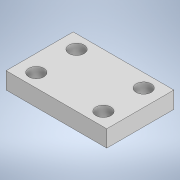
# Autodesk Inventor part: beltpress
Saved by Autodesk Inventor 2020.2 (Build 242310000, 310)
## iProperties
Created: 2020-08-07
Part Number: beltpress
Material: Generic
Document SubType Name: Modeling
Designer: JK
Density: 1 g/cm^3
Appearance: Default
Author: JK
Autodesk Inventor part; units mm, degrees
ref_plane "YZ Plane" through (0, 0, 0) normal (1, 0, 0) x (0, 1, 0)
ref_plane "XZ Plane" through (0, 0, 0) normal (0, 1, 0) x (-1, 0, 0)
ref_plane "XY Plane" through (0, 0, 0) normal (0, 0, 1) x (1, 0, 0)
sketch "Sketch1" plane through (0, 0, 0) normal (0, 1, 0) x (-1, 0, 0)
  line L0 (445.6248, 255.5836) -> (415.6248, 255.5836)
  line L1 (415.6248, 255.5836) -> (415.6248, 235.5836)
  line L2 (415.6248, 235.5836) -> (445.6248, 235.5836)
  line L3 (445.6248, 235.5836) -> (445.6248, 255.5836)
  circle A0 centre (440.6248, 251.5836) radius 2.25
  circle A1 centre (440.6248, 239.5836) radius 2.25
  circle A2 centre (420.6248, 251.5836) radius 2.25
  circle A3 centre (420.6248, 239.5836) radius 2.25
  dimension "d8" = 4.5
  dimension "d9" = 20
  dimension "d10" = 30
  dimension "d11" = 20
  dimension "d12" = 12
  dimension "d13" = 4
  dimension "d14" = 5
  constraints: 8 end point, 4 centre point, 3 equal radius, 2 horizontal alignment, 2 parallel, 2 vertical alignment, 1 horizontal, 1 perpendicular
  measures "d8" diameter of A0
  measures "d9" distance of L2.end L0.start
  measures "d10" distance of L1.end L2.end
  measures "d11" distance of A2.centre A0.centre
  measures "d12" distance of A0.centre A1.centre
  measures "d13" distance from line of A0.centre L0
  measures "d14" distance from line of A2.centre L1
extrude "Extrusion1" add sketch "Sketch1" along normal blind 5
body "Solid1"
